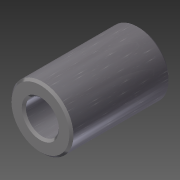
# Autodesk Inventor part: BearingLinearLMU8
Saved by Autodesk Inventor 2015 SP1 (Build 190203100, 203)
## iProperties
Category: Hardware
Created: 2014-08-25
Part Number: BearingLinearLMU8
Material: Steel, Alloy
Document SubType Name: Modeling
Designer: t_clevj
Density: 7.73 g/cm^3
Appearance: Semi-Polished
Mass: 23.3192 g
Surface Area: 19.4473 cm^2
Volume: 3.01671 cm^3
Vendor: Misumi
Catalog Web Link: http://us.misumi-ec.com/vona2/detail/110300026540/
Author: t_clevj
Title: Bearing Linear LMU8
Autodesk Inventor part; units mm, degrees
ref_plane "YZ Plane" through (0, 0, 0) normal (1, 0, 0) x (0, 1, 0)
ref_plane "XZ Plane" through (0, 0, 0) normal (0, 1, 0) x (-1, 0, 0)
ref_plane "XY Plane" through (0, 0, 0) normal (0, 0, 1) x (1, 0, 0)
sketch "Sketch1" plane through (0, 0, 0) normal (0, 1, 0) x (-1, 0, 0)
  circle A0 centre (0, 0) radius 4
  circle A1 centre (0, 0) radius 7.5
  dimension "d0" = 8
  dimension "d1" = 15
  constraints: 2 centre point, 2 coincident
  measures "d0" diameter of A0
  measures "d1" diameter of A1
extrude "Extrusion1" add sketch "Sketch1" along normal blind 24
chamfer "Chamfer1" distance 0.5 angle 45 4 edges at (7.5, 24, 0) (4, 24, 0) (7.5, 0, 0) (4, 0, 0)
body "Solid1"
